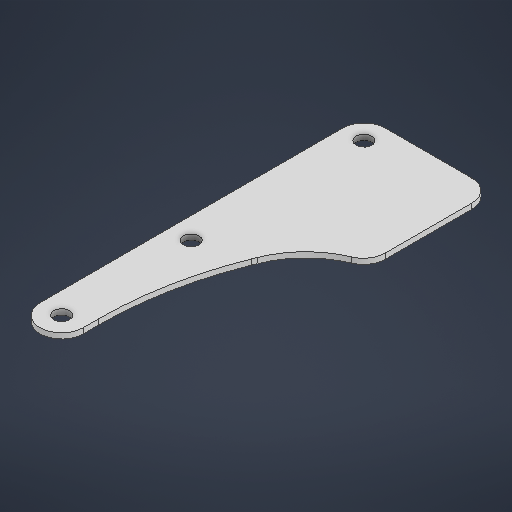
# Autodesk Inventor part: Lady Brown Tab Top
Saved by Autodesk Inventor 2025 (Build 290162000, 162)
## iProperties
Created: 2024-12-29
Part Number: Lady Brown Tab Top
Material: Generic
Document SubType Name: Modeling
Designer: Juan
Density: 1 g/cm^3
Appearance: Default
Author: Juan
Autodesk Inventor part; units mm, degrees
ref_plane "YZ Plane" through (0, 0, 0) normal (1, 0, 0) x (0, 1, 0)
ref_plane "XZ Plane" through (0, 0, 0) normal (0, 1, 0) x (-1, 0, 0)
ref_plane "XY Plane" through (0, 0, 0) normal (0, 0, 1) x (1, 0, 0)
sketch "Sketch1" plane through (0, 0, 0) normal (0, 1, 0) x (-1, 0, 0)
  circle A0 centre (0, 0) radius 2.3241
  line L0 (0, 0) -> (0, -63.5)
  circle A1 centre (0, -63.5) radius 2.3241
  line L1 (0, 0) -> (0, -63.5) construction
  line L2 (-6.35, 0) -> (-6.35, -63.5)
  line L3 (6.35, -63.5) -> (6.35, 0)
  arc A2 (6.35, 0) -> (-6.35, 0) centre (0, 0) ccw
  arc A3 (-6.35, -63.5) -> (6.35, -63.5) centre (0, -63.5) ccw
  line L4 (0, -63.5) -> (-15.9411, -63.5) construction
  line L5 (0, -57.15) -> (-15.9411, -57.15)
  line L6 (-15.9411, -69.85) -> (0, -69.85)
  arc A4 (0, -69.85) -> (0, -57.15) centre (0, -63.5) ccw
  arc A5 (-15.9411, -57.15) -> (-15.9411, -69.85) centre (-15.9411, -63.5) ccw
  line L7 (0, -63.5) -> (-25.4, -63.5) construction
  line L8 (0, -57.15) -> (-25.4, -57.15)
  line L9 (-25.4, -69.85) -> (0, -69.85)
  arc A6 (0, -69.85) -> (0, -57.15) centre (0, -63.5) ccw
  arc A7 (-25.4, -57.15) -> (-25.4, -69.85) centre (-25.4, -63.5) ccw
  line L10 (-5.9094, 2.3241) -> (-31.2958, -61.1417)
  line L11 (-25.4, -63.5) -> (-25.4, -37.9561) construction
  line L12 (-19.05, -63.5) -> (-19.05, -37.9561)
  line L13 (-31.75, -37.9561) -> (-31.75, -63.5)
  arc A8 (-31.75, -63.5) -> (-19.05, -63.5) centre (-25.4, -63.5) ccw
  arc A9 (-19.05, -37.9561) -> (-31.75, -37.9561) centre (-25.4, -37.9561) ccw
  line L14 (-27.3182, -31.9028) -> (-18.4799, -29.102)
  point P0 (0, -31.75)
  point P1 (-7.9706, -63.5)
  point P2 (-22.0988, -61.949)
  point P3 (-12.7, -63.5)
  point P4 (-6.35, -57.15)
  point P5 (-25.4, -50.7281)
  dimension "d0" = 4.6482
  dimension "d1" = 63.5
  dimension "d2" = 4.6482
  dimension "d3" = 12.7
  dimension "d6" = 15.9411
  dimension "d7" = 25.4
  constraints: 38 end point, 20 point on circle, 18 tangent, 10 centre point, 5 equal length, 4 midpoint, 2 coincident, 2 point on line, 2 vertical, 1 perpendicular
  measures "d0" diameter of A0
  measures "d1" distance of L0.start L0.end
  measures "d2" diameter of A1
  measures "d3" diameter of A3
  measures "d6" distance of L1.end L4.end
  measures "d7" distance of L1.end L7.end
extrude "Extrusion2" add sketch "Sketch1" along normal blind 1.5875 contours L5 L2 A2 L3 A4 | A4 A3 L2 L5 | L5 L8 L12 A9 L10 A2 L2 | L2 A3 L6 A5 A8 L12 L5 | A5 L12 L8 | L12 A8 A5 | A5 A8 A7 L8 L12 | L8 A7 L10 A9 L12 | L9 A8 A5
extrude "Extrusion3" add sketch "Sketch1" along normal blind 1.5875 contours L10 A9 L14 | L10 A7 L13 A9
fillet "Fillet1" radius 25.4 1 edges at (18.4799, 0.7937, -29.102)
sketch "Sketch2" plane through (0, 1.5875, 0) normal (0, 1, 0) x (1, 0, 0)
  circle A0 centre (0, 0) radius 2.3241 projected
  line L0 (0, 0) -> (0, -25.4)
  line L1 (0, -25.4) -> (0, 0) construction
  line L2 (6.35, -25.4) -> (6.35, 0)
  line L3 (-6.35, 0) -> (-6.35, -25.4)
  arc A1 (-6.35, -25.4) -> (6.35, -25.4) centre (0, -25.4) ccw
  arc A2 (6.35, 0) -> (-6.35, 0) centre (0, 0) ccw
  circle A3 centre (0, -25.4) radius 2.3241
  line L4 (0, 0) -> (0, 12.6898)
  circle A4 centre (0, 12.6898) radius 2.3241
  point P0 (0, -12.7)
  dimension "d13" = 25.4
  dimension "d17" = 4.6482
  dimension "d20" = 4.6482
  constraints: 12 end point, 4 centre point, 4 point on circle, 4 tangent, 2 coincident, 2 equal length, 1 midpoint, 1 point on line, 1 vertical
  measures "d13" distance of L0.start L0.end
  measures "d17" diameter of A3
  measures "d20" diameter of A4
extrude "Extrusion4" add sketch "Sketch2" against normal blind 1.5875 contours A0 L0 L4 | A3 | A2 L2 A1 L3 | L4 L0 A0
fillet "Fillet2" radius 101.6 1 edges at (6.35, 0.7937, 1.2226)
extrude "Extrusion5" cut sketch "Sketch2" against normal blind 1.5875 contours A3
extrude "Extrusion6" cut sketch "Sketch2" against normal blind 1.5875 contours A4
body "Solid2"
